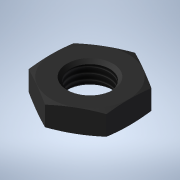
# Autodesk Inventor part: DIN-439-B - M10x1.25(F)
Saved by Autodesk Inventor 2021 (Build 250183000, 183)
## iProperties
Created: 2025-06-06
Part Number: DIN-439-B - M10x1.25(F)
Material: Generic
Catalog Web Link: www.cadenas.de
Description: DIN-439 Form B-Hex nut
Vendor: FESTO
Document SubType Name: Modeling
Designer: psAdmin
Manufacturer: FESTO
Mass: 0.939092 g
Surface Area: 7.79069 cm^2
Volume: 0.939092 cm^3
Density: 1 g/cm^3
Appearance: PSOLRGB-175-175-175
Category: PARTsolutions
Company: FESTO
Title: DIN-439-B - M10x1.25
Author: Cadenas PARTsolutions
Comments: Hex nut
PSOL_IDENT_0: {$CADENAS_DATA/23d-libs/festo/zyl_zubeh/din_439_b/din_439_form_b.prj},192 {VTYP=3D},{NB=DIN-439-B -
PSOL_IDENT_1: M10x1.25(F)},{LINA=DIN-439-B - M10x1.25},{NN=DIN-439 Form B},{DATE=28.05.2015 11:05:12},{GEOMDATE=28
PSOL_IDENT_2: .05.2015 08:07:00},{VERSION=},{LINEID=110},{WBVAR=},{WBNUMERIC=}  {NB=DIN-439-B - M10x1.25(F)},{LINA=
PSOL_IDENT_3: DIN-439-B - M10x1.25},{KT=X},{IDNR=},{NENN=M10x1.25},{DG=10.000},{DK=8.647},{M=5.000},{S=17.000},{P=
PSOL_IDENT_4: 1.250}
NB: DIN-439-B - M10x1.25(F)
NN: DIN-439 Form B
NT: Hex nut
NBSYN: DIN-439-B - $NENN.(F)
LINA: DIN-439-B - M10x1.25
CATALOG: Festo
ROWDESC: M10x1.25
NENN: M10x1.25
DG: 10
DK: 8.647
M: 5
S: 17
P: 1.25
SUPPLIER: FESTO
ARTICLENO: DIN-439-B - M10x1.25(F)
BOMINFO: DIN-439-B - M10x1.25
CREATOR: CADENAS GmbH
Autodesk Inventor part; units mm, degrees
ref_plane "YZ Plane" through (0, 0, 0) normal (1, 0, 0) x (0, 1, 0)
ref_plane "XZ Plane" through (0, 0, 0) normal (0, 1, 0) x (-1, 0, 0)
ref_plane "XY Plane" through (0, 0, 0) normal (0, 0, 1) x (1, 0, 0)
sketch "Sketch_1" plane through (0, 0, 0) normal (0, 0, 1) x (1, 0, 0)
  line L0 (0, -5) -> (0, 0)
  line L1 (0, 0) -> (8.45, 0)
  line L2 (8.45, 0) -> (17.7801, -2.5)
  line L3 (17.7801, -2.5) -> (8.45, -5)
  line L4 (8.45, -5) -> (0, -5)
  line L5 (0, -5) -> (0, 0)
  constraints: 12 end point
revolve "Revolution1" add sketch "Sketch_1" angle 360 about axis through (0, -5, 0) along (0, 1, 0)
sketch "Sketch_2" plane through (0, 0, 0) normal (0, 1, 0) x (-1, 0, 0)
  line L0 (34, -34) -> (34, 34)
  line L1 (34, 34) -> (-34, 34)
  line L2 (-34, 34) -> (-34, -34)
  line L3 (-34, -34) -> (34, -34)
  line L4 (8.5, 4.9075) -> (0, 9.815)
  line L5 (0, 9.815) -> (-8.5, 4.9075)
  line L6 (-8.5, 4.9075) -> (-8.5, -4.9075)
  line L7 (-8.5, -4.9075) -> (0, -9.815)
  line L8 (0, -9.815) -> (8.5, -4.9075)
  line L9 (8.5, -4.9075) -> (8.5, 4.9075)
  constraints: 20 end point
extrude "Extrusion1" cut sketch "Sketch_2" along normal mid plane 12
sketch "Sketch_3" plane through (0, 0, 0) normal (0, 0, 1) x (1, 0, 0)
  line L0 (0, -5) -> (0, 0)
  line L1 (0, 0) -> (5, 0)
  line L2 (5, 0) -> (4.3235, -0.6765)
  line L3 (4.3235, -0.6765) -> (4.3235, -4.3235)
  line L4 (4.3235, -4.3235) -> (5, -5)
  line L5 (5, -5) -> (0, -5)
  line L6 (0, -5) -> (0, 0)
  constraints: 14 end point
revolve "Revolution2" cut sketch "Sketch_3" angle 360 about axis through (0, -5, 0) along (0, -1, 0)
thread "Thread1" size "M10x1.25" class "6H" standard "ISO Metric profile" full length
ref_plane "2CYL_XY" through (0, -2.5, 0) normal (0, 1, 0) x (1, 0, 0)
ref_plane "2CYL_YZ" through (0, -2.5, 0) normal (1, 0, 0) x (0, 0, -1)
ref_plane "2CYL_ZX" through (0, -2.5, 0) normal (0, 0, -1) x (0, 1, 0)
ref_plane "din439b_punkt_XY" through (0, 0, 0) normal (0, 1, 0) x (1, 0, 0)
ref_plane "din439b_punkt_YZ" through (0, 0, 0) normal (1, 0, 0) x (0, 0, -1)
ref_plane "din439b_punkt_ZX" through (0, 0, 0) normal (0, 0, -1) x (0, 1, 0)
body "Solid1"
